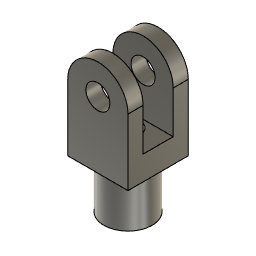
Exercise_2 v1 (Autodesk Fusion 360 design; units mm, degrees)
Autodesk Fusion 360 part; units mm, degrees
sketch "Sketch1" plane through (0, 0, 0) normal (0, 0, 1) x (1, 0, 0)
  circle A0 centre (0, 0) radius 10
  line L0 (-12.5, 12.5) -> (12.5, 12.5)
  line L1 (12.5, 12.5) -> (12.5, -12.5)
  line L2 (12.5, -12.5) -> (-12.5, -12.5)
  line L3 (-12.5, -12.5) -> (-12.5, 12.5)
  line L4 (-12.5, 6.25) -> (12.5, 6.25)
  line L5 (12.5, 6.25) -> (12.5, -6.25)
  line L6 (12.5, -6.25) -> (-12.5, -6.25)
  line L7 (-12.5, -6.25) -> (-12.5, 6.25)
  circle A1 centre (0, 0) radius 5
  dimension "d1" = 20
  dimension "d2" = 25
  dimension "d3" = 25
  dimension "d4" = 12.5
  dimension "d5" = 12.5
  dimension "d6" = 25
  dimension "d7" = 12.5
  dimension "d8" = 6.25
  dimension "d9" = 10
  constraint coincident A0.centre A1.centre
  constraint horizontal L0
  constraint vertical L1
  constraint horizontal L2
  constraint vertical L3
  constraint horizontal L4
  constraint vertical L5
  constraint horizontal L6
  constraint vertical L7
  constraint coincident L3 L4.start
  constraint concentric A0 A1
  measures "d1" diameter of A0
  measures "d2" distance of L0.start L0.end
  measures "d3" distance of L0.end L1.end
  measures "d4" distance of A0.centre L2
  measures "d5" distance of A0.centre L1
  measures "d6" distance of L4.start L4.end
  measures "d7" distance of L4.end L5.end
  measures "d8" distance of L2 L5.end
  measures "d9" diameter of A1
extrude "Extrude1" add sketch "Sketch1" along normal blind 40 contours A0 L4 | A0 L0 L1 L3 L4 | A0 L1 L2 L3 L6 | A0 L6 makes body 1 at (-4.1667, 6.25, 13.3333) makes body 2 at (4.1667, -6.25, 13.3333)
extrude "Extrude2" add sketch "Sketch1" against normal blind 20 contours A0 L4 L6 | A0 L4 | A0 L6 bodies 1 2
extrude "Extrude3" add sketch "Sketch1" along normal blind 10 contours A0 L4 L6 | A0 L1 L4 L5 L6 | A0 L3 L4 L6 L7 bodies 1
sketch "Sketch2" plane through (0, 12.5, 0) normal (0, 1, 0) x (-1, 0, 0)
  line L0 (-12.5, 0) -> (12.5, 0)
  line L1 (12.5, 0) -> (12.5, 40)
  line L2 (12.5, 40) -> (-12.5, 40)
  line L3 (-12.5, 40) -> (-12.5, 0)
  circle A0 centre (0, 27.5) radius 5
  line L4 (12.5, 0) -> (-12.5, 0)
  dimension "d16" = 10
  dimension "d17" = 27.5
  measures "d16" diameter of A0
  measures "d17" distance of A0.centre L4
extrude "Extrude4" cut sketch "Sketch2" against normal up to surface (25 mm away) contours A0 bodies 1
fillet "Fillet1" radius 12.5 4 edges at (12.5, 9.375, 40) (-12.5, 9.375, 40) (-12.5, -9.375, 40) (12.5, -9.375, 40) on bodies 1
equation "d4 = ( 25 / 2 ) * 1 mm"
equation "d5 = ( 25 / 2 ) * 1 mm"
equation "d8 = ( 12.5 / 2 ) * 1 mm"
